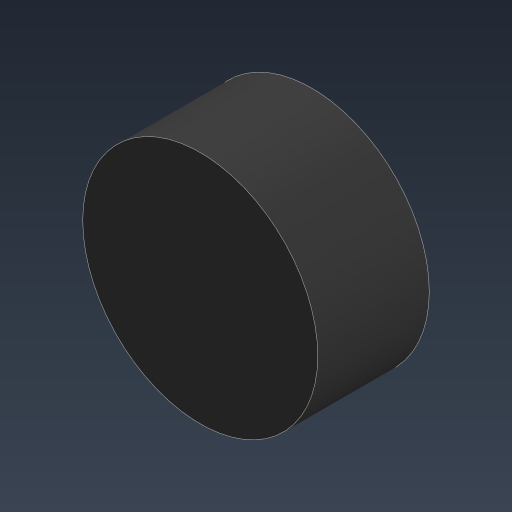
# Autodesk Inventor part: oponka
Saved by Autodesk Inventor 2023 (Build 270158000, 158)
## iProperties
Created: 2025-04-29
Part Number: oponka
Material: Rubber, Silicone
Document SubType Name: Modeling
Designer: szymo
Density: 1.25 g/cm^3
Appearance: Rubber - Black
Mass: 22.8201 g
Surface Area: 40.1064 cm^2
Volume: 18.2561 cm^3
Author: szymo
Autodesk Inventor part; units mm, degrees
ref_plane "YZ Plane" through (0, 0, 0) normal (1, 0, 0) x (0, 1, 0)
ref_plane "XZ Plane" through (0, 0, 0) normal (0, 1, 0) x (-1, 0, 0)
ref_plane "XY Plane" through (0, 0, 0) normal (0, 0, 1) x (1, 0, 0)
sketch "Sketch1" plane through (0, 0, 0) normal (0, 0, 1) x (1, 0, 0)
  circle A0 centre (-1.7398, 4.8953) radius 7.9323
  circle A1 centre (-1.7398, 4.8953) radius 20
  circle A2 centre (5.4482, 9.0453) radius 1 projected
  circle A3 centre (-8.9278, 9.0453) radius 1 projected
  arc A4 (-11.3542, 2.1453) -> (7.8747, 2.1453) centre (-1.7398, 4.8953) ccw projected
  arc A5 (6.799, 0.7313) -> (6.6562, 2.1453) centre (5.5856, 1.323) ccw projected
  line L0 (6.6562, 2.1453) -> (7.8747, 2.1453) projected
  line L1 (-11.3542, 2.1453) -> (-10.1358, 2.1453) projected
  arc A6 (-10.1358, 2.1453) -> (-10.2785, 0.7313) centre (-9.0651, 1.323) ccw projected
  arc A7 (-10.2785, 0.7313) -> (-5.9038, -3.6435) centre (-1.7398, 4.8953) ccw projected
  arc A8 (-5.9038, -3.6435) -> (-4.7204, -1.2166) centre (-5.3121, -2.43) ccw projected
  arc A9 (-4.7204, -1.2166) -> (1.2408, -1.2166) centre (-1.7398, 4.8953) ccw projected
  arc A10 (1.2408, -1.2166) -> (2.4243, -3.6435) centre (1.8325, -2.43) ccw projected
  arc A11 (2.4243, -3.6435) -> (6.799, 0.7313) centre (-1.7398, 4.8953) ccw projected
  point P0 (0, 0)
  point P1 (-9.6144, 5.85)
  point P2 (-8.9278, 8.0453)
  point P3 (5.4482, 8.0453)
  dimension "d0" = 40
  constraints: 2 coincident, 2 vertical alignment, 1 centre point, 3 other
  measures "d0" diameter of A1
ref_plane "Work Plane1" through (-9.6144, -3.5, -18.975) normal (0, 0, -1) x (0, 1, 0)
extrude "Extrusion1" add sketch "Sketch1" against normal up to surface (18.975 mm away) contours A0 A10 A9 A8 A3 A2 | A2 A0 | A0 A2 | A10 A11 A5 L0 A4 L1 A6 A7 A8 A0 | A0 A8 A9 A10 | A3 A0 | A0 A3 | A1
body "Solid1"
